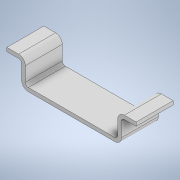
# Autodesk Inventor part: din_rail
Saved by Autodesk Inventor 2020.1 (Build 241239000, 239)
## iProperties
Created: 2020-01-18
Part Number: din_rail
Material: Generic
Document SubType Name: Modeling
Designer: yusaku
Density: 1 g/cm^3
Appearance: Default
Author: yusaku
Autodesk Inventor part; units mm, degrees
ref_plane "YZ Plane" through (0, 0, 0) normal (1, 0, 0) x (0, 1, 0)
ref_plane "XZ Plane" through (0, 0, 0) normal (0, 1, 0) x (-1, 0, 0)
ref_plane "XY Plane" through (0, 0, 0) normal (0, 0, 1) x (1, 0, 0)
sketch "Sketch1" plane through (0, 0, 0) normal (0, 0, 1) x (1, 0, 0)
  line L0 (0, 0) -> (11.7, 0)
  arc A0 (11.7, 0) -> (13.5, 1.8) centre (11.7, 1.8) ccw
  line L1 (13.5, 1.8) -> (13.5, 5.7)
  arc A1 (14.3, 6.5) -> (13.5, 5.7) centre (14.3, 5.7) ccw
  line L2 (14.3, 6.5) -> (17.5, 6.5)
  line L3 (17.5, 6.5) -> (17.5, 7.5)
  line L4 (17.5, 7.5) -> (14.3, 7.5)
  arc A2 (14.3, 7.5) -> (12.5, 5.7) centre (14.3, 5.7) ccw
  line L5 (12.5, 5.7) -> (12.5, 1.8)
  arc A3 (11.7, 1) -> (12.5, 1.8) centre (11.7, 1.8) ccw
  line L6 (11.7, 1) -> (0, 1)
  line L7 (0, 1) -> (0, 0)
  dimension "d0" = 1
  dimension "d2" = 0.8
  dimension "d3" = 25
  dimension "d4" = 35
  dimension "d5" = 7.5
  constraints: 16 end point, 8 point on circle, 8 tangent, 7 perpendicular, 4 centre point, 2 concentric, 1 equal radius, 1 horizontal
  measures "d0" distance of L6.end L0.start
  measures "d2" radius of A3
  measures "d3" diameter of L5 L7
  measures "d4" diameter of L3 L7
  measures "d5" distance between parallel lines of L4 L0
extrude "Extrusion1" add sketch "Sketch1" along normal blind 10
mirror "Mirror1" about plane through (0, 1, 0) normal (-1, 0, 0) of "Extrusion1"
body "Solid1"
